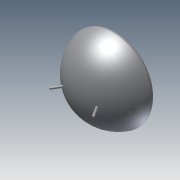
# Autodesk Inventor part: head
Saved by Autodesk Inventor 2011 (Build 150239000, 239)
## iProperties
Created: 2013-01-27
Part Number: head
Document SubType Name: Modeling
Designer: bot_m8ker
Density: 1 g/cm^3
Author: bot_m8ker
Autodesk Inventor part; units mm, degrees
ref_plane "YZ Plane" through (0, 0, 0) normal (1, 0, 0) x (0, 1, 0)
ref_plane "XY Plane" through (0, 0, 0) normal (0, 0, 1) x (1, 0, 0)
sketch "Sketch1" plane through (0, 0, 0) normal (0, 0, 1) x (1, 0, 0)
  circle A0 centre (0, 0) radius 12.7
  line L0 (-19.05, 0) -> (19.05, 0)
  dimension "d0" = 25.4
  dimension "d1" = 38.1
  constraints: 2 coincident, 2 end point, 1 centre point, 1 horizontal, 1 midpoint
  measures "d0" diameter of A0
  measures "d1" distance of L0.start L0.end
extrude "Extrusion1" add sketch "Sketch1" along normal blind 12.7
fillet "Fillet1" radius 12.7 1 edges at (-12.7, 0, 12.7)
move faces "Move Face1" translate (0, 0, -3.175) faces at (12.6588, -1.0219, 0.0001) (-4.3479, -11.7815, 1.8929) (0, 0, 12.7)
fillet "Fillet2" radius 0.9525 1 edges at (-12.2967, -0.0008, 0)
ref_plane "Work Plane1" through (0, -11.43, 0) normal (0, 1, 0) x (-1, 0, 0)
sketch "Sketch3" plane through (0, -11.43, 0) normal (0, 1, 0) x (-1, 0, 0)
  circle A0 centre (4.1275, 4.445) radius 1.1112
  circle A1 centre (-4.1275, 4.445) radius 1.1112
  point P0 (0, 0)
  dimension "d8" = 4.1275
  dimension "d9" = 4.1275
  dimension "d10" = 4.445
  dimension "d11" = 4.445
  dimension "d37" = 2.2225
  dimension "d38" = 2.2225
  constraints: 2 centre point
  measures "d8" horizontal distance of point (0, 0) A0.centre
  measures "d9" horizontal distance of A1.centre point (0, 0)
  measures "d10" vertical distance of point (0, 0) A0.centre
  measures "d11" vertical distance of point (0, 0) A1.centre
  measures "d37" diameter of A0
  measures "d38" diameter of A1
hole "Hole1" at (-4.1275, -11.43, 4.445) at (4.1275, -11.43, 4.445) direction (0, 1, 0) diameter 1.5875 depth 19.05
sketch "Sketch4" plane through (0, 0, 0) normal (0, 1, 0) x (-1, 0, 0)
  line L0 (0.275, -0.1587) -> (0, 0)
  line L1 (0, 0) -> (6.35, 10.9985)
  line L2 (6.35, 10.9985) -> (6.625, 10.8398)
  line L3 (6.625, 10.8398) -> (0.275, -0.1587)
  line L4 (0, 0) -> (-0.275, -0.1587)
  line L5 (-0.275, -0.1587) -> (-9.8, 16.339)
  line L6 (-9.8, 16.339) -> (-9.525, 16.4978)
  line L7 (-9.525, 16.4978) -> (0, 0)
  dimension "d19" = 12.7
  dimension "d20" = 0.3175
  dimension "d21" = 19.05
  dimension "d22" = 0.3175
  constraints: 16 end point, 4 parallel, 2 perpendicular, 1 coincident
  measures "d19" distance of L2.end L0.start
  measures "d20" distance of L1.end L2.end
  measures "d21" distance of L4.end L5.end
  measures "d22" distance of L5.end L6.end
revolve "Revolution1" add sketch "Sketch4" angle 360 about axis through (0, 0, 0) along (-0.5, 0, 0.8660254) contours L0 L1 L2 L3
fillet "Fillet3" radius 0.3175 1 edges at (-6.075, 0, 11.1573)
sketch "Sketch5" plane through (0, 0, 0) normal (0, 1, 0) x (-1, 0, 0)
  line L0 (0, 0) -> (-0.275, -0.1588)
  line L1 (-0.275, -0.1588) -> (-6.625, 10.8398)
  line L2 (-6.625, 10.8398) -> (-6.35, 10.9985)
  line L3 (-6.35, 10.9985) -> (0, 0)
  dimension "d25" = 12.7
  dimension "d26" = 0.3175
  constraints: 8 end point, 2 parallel, 1 coincident, 1 perpendicular
  measures "d25" distance of L0.end L1.end
  measures "d26" distance of L1.end L2.end
revolve "Revolution2" add sketch "Sketch5" angle 360 about axis through (6.35, 0, 10.9985) along (-0.5, 0, -0.8660254)
fillet "Fillet4" radius 0.3175 1 edges at (6.075, 0, 11.1573)
sketch "Sketch6" plane through (0, 0, 0) normal (0, 1, 0) x (-1, 0, 0)
  circle A0 centre (4.1275, 4.445) radius 0.7937
  circle A1 centre (-4.1275, 4.445) radius 0.7937
  point P0 (0, 0)
  dimension "d30" = 4.445
  dimension "d31" = 4.1275
  dimension "d32" = 4.1275
  dimension "d33" = 1.5875
  dimension "d34" = 1.5875
  constraints: 2 centre point, 1 horizontal alignment
  measures "d30" vertical distance of point (0, 0) A0.centre
  measures "d31" horizontal distance of point (0, 0) A0.centre
  measures "d32" horizontal distance of A1.centre point (0, 0)
  measures "d33" diameter of A0
  measures "d34" diameter of A1
extrude "Extrusion2" add sketch "Sketch6" against normal blind 0.254
body "Solid1"
